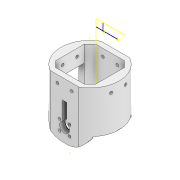
# Autodesk Inventor part: brazo_base_salvaculos.pt
Saved by Autodesk Inventor 2021 (Build 250183000, 183)
## iProperties
Created: 2021-03-15
Part Number: brazo_base_salvaculos.pt
Material: Plástico ABS
Document SubType Name: Modeling
Designer: Joaquín
Density: 1.06 g/cm^3
Appearance: Suave - Blanco
Author: Joaquín
Autodesk Inventor part; units mm, degrees
ref_plane "YZ Plane" through (0, 0, 0) normal (1, 0, 0) x (0, 1, 0)
ref_plane "XZ Plane" through (0, 0, 0) normal (0, 1, 0) x (-1, 0, 0)
ref_plane "XY Plane" through (0, 0, 0) normal (0, 0, 1) x (1, 0, 0)
sketch "Boceto4" plane through (0, 0, 0) normal (0, 1, 0) x (-1, 0, 0)
  line L0 (-22.5, 0) -> (-22.5, -16)
  line L1 (0, -22.5) -> (-16, -22.5)
  line L2 (-16, -22.5) -> (-22.5, -16)
  line L3 (0, -22.5) -> (16, -22.5)
  line L4 (22.5, 0) -> (22.5, -16)
  line L5 (22.5, -16) -> (16, -22.5)
  line L6 (22.5, 0) -> (22.5, 16)
  line L7 (0, 22.5) -> (16, 22.5)
  line L8 (16, 22.5) -> (22.5, 16)
  line L9 (0, 22.5) -> (-16, 22.5)
  line L10 (-22.5, 0) -> (-22.5, 16)
  line L11 (-22.5, 16) -> (-16, 22.5)
  line L12 (-16, 25) -> (16, 25)
  line L13 (25, 16) -> (25, -16)
  line L14 (16, -25) -> (-16, -25)
  line L15 (-25, -16) -> (-25, 16)
  line L16 (16, -25) -> (25, -16)
  line L17 (25, 16) -> (16, 25)
  line L18 (-25, 16) -> (-16, 25)
  line L19 (-25, -16) -> (-16, -25)
  point P0 (0, 0)
  dimension "d22" = 360
  constraints: 40 end point, 3 parallel, 1 horizontal, 1 perpendicular, 29 other
extrude "Extrusión2" add sketch "Boceto4" along normal blind 100
sketch "Boceto5" plane through (0, 0, 0) normal (0, -1, 0) x (1, 0, 0)
  circle A0 centre (0, 0) radius 32.5
  line L0 (-25, -16) -> (-25, 16) projected
  line L1 (-25, 16) -> (-16, 25) projected
  line L2 (-25, 16) -> (-16, 25)
  line L3 (-16, 25) -> (16, 25)
  line L4 (16, 25) -> (25, 16) projected
  line L5 (16, 25) -> (25, 16)
  line L6 (25, 16) -> (25, -16) projected
  line L7 (25, 16) -> (25, -16)
  line L8 (25, -16) -> (16, -25)
  line L9 (16, -25) -> (-16, -25) projected
  line L10 (16, -25) -> (-16, -25)
  line L11 (-16, -25) -> (-25, -16)
  line L12 (-25, -16) -> (-25, 16)
  constraints: 16 end point, 6 equal length, 1 centre point, 1 coincident, 1 horizontal, 1 perpendicular
sketch "Boceto7" plane through (-16, 0, 25) normal (0, 0, 1) x (1, 0, 0)
  line L0 (-9, 18) -> (-1.4121, 2.8243)
  line L1 (41, 0) -> (41, 100) projected
  line L2 (32, 0) -> (32, 100) projected
  line L3 (33.4121, 2.8243) -> (41, 18)
  line L4 (-9, 0) -> (-9, 100) projected
  line L5 (-19, 18) -> (-19, 0)
  line L6 (51, 18) -> (51, 0)
  line L7 (-9, 0) -> (-9, 10)
  line L8 (-9, 0) -> (-9, 100) projected
  line L9 (41, 0) -> (41, 10)
  line L10 (41, 10) -> (-9, 10)
  line L11 (-9, 10) -> (16, 10)
  ellipse E0 centre (16, 10) end of major axis (-9, 10) minor radius 10 (-1.4121, 2.8243) -> (33.4121, 2.8243) ccw
  line L12 (0, 0) -> (0, 100) projected
  line L13 (-19, 0) -> (16, 0)
  line L14 (16, 0) -> (51, 0)
  line L15 (32, 0) -> (0, 0) projected
  line L16 (-19, 18) -> (-19, 38)
  line L17 (51, 18) -> (51, 38)
  arc A0 (-19, 38) -> (-9, 18) centre (10.8998, 40.4499) ccw
  arc A1 (41, 18) -> (51, 38) centre (21.1002, 40.4499) ccw
  point P0 (32, 2.3163)
  dimension "d53" = 10
  dimension "d54" = 10
  dimension "d55" = 25
  dimension "d58" = 20
  dimension "d59" = 20
  dimension "d60" = 30
  dimension "d61" = 30
  constraints: 24 end point, 4 point on circle, 4 point on line, 2 centre point, 2 horizontal, 2 vertical, 1 coincident, 1 collinear, 1 midpoint, 5 other
  measures "d53" distance of L7.end L4.start
  measures "d54" distance of L1.start L9.end
  measures "d55" distance of L7.end L11.end
  measures "d58" distance of L5.start L16.end
  measures "d59" distance of L6.start L17.end
  measures "d60" radius of A0
  measures "d61" radius of A1
extrude "Extrusión4" add sketch "Boceto5" against normal blind 100
extrude "Extrusión8" cut sketch "Boceto7" against normal mid plane 200 contours L0 L10 L4 | L4 L13 L5 L16 A0 | L0 E0 L12 L13 L4 L10 | E0 L13 L12 | E0 L2 L14 | E0 L3 L10 L1 L14 L2 | L3 L1 L10 | L1 A1 L17 L6 L14
sketch "Boceto10" plane through (-16, 100, -22.5) normal (0, 0, 1) x (1, 0, 0)
  line L0 (0, 0) -> (8, 0)
  line L1 (0, 0) -> (32, 0) projected
  line L2 (8, 0) -> (8, -8)
  circle A0 centre (8, -8) radius 1.5
  line L3 (32, -97.6837) -> (32, 0) projected
  line L4 (32, 0) -> (24, 0)
  line L5 (24, 0) -> (24, -8)
  circle A1 centre (24, -8) radius 1.5
  point P0 (16, -100)
  dimension "d95" = 8
  dimension "d96" = 8
  dimension "d97" = 3
  dimension "d98" = 8
  dimension "d99" = 8
  dimension "d100" = 3
  constraints: 8 end point, 2 centre point, 2 coincident, 2 perpendicular, 2 point on line
  measures "d95" distance of L0.start L0.end
  measures "d96" distance of L0.end L2.end
  measures "d97" diameter of A0
  measures "d98" distance of L1.end L4.end
  measures "d99" distance of L4.end L5.end
  measures "d100" diameter of A1
extrude "Extrusión12" cut sketch "Boceto10" along normal mid plane 200
sketch "Boceto11" plane through (22.5, 100, -16) normal (-1, 0, 0) x (0, 0, 1)
  circle A0 centre (8, -8) radius 1.5
  circle A1 centre (24, -8) radius 1.5
  point P0 (16, -100)
  point P1 (0, 0)
  point P2 (32, 0)
  constraints: 2 centre point
extrude "Extrusión13" cut sketch "Boceto11" against normal mid plane 200
sketch "Boceto14" plane through (0, 100, 0) normal (0, 1, 0) x (1, 0, 0)
  point P0 (0, 0)
sketch "Boceto15" plane through (-16, 100, -22.5) normal (0, 0, 1) x (1, 0, 0)
  line L0 (13, -81) -> (10, -81) projected
  line L1 (22, -69) -> (19, -69) projected
  arc A0 (32, -94.1587) -> (0, -94.1587) centre (16, -75.1663) ccw
  circle A1 centre (16, -75.1663) radius 20
  line L2 (0, -97.6837) -> (0, 0) projected
  line L3 (0, -87.1663) -> (0, -97.6837)
  line L4 (32, -97.6837) -> (32, 0) projected
  line L5 (32, -87.1663) -> (32, -97.6837)
  ellipse E0 centre (16, -90) end of major axis (41, -90) minor radius 10 (-1.4121, -97.1757) -> (0, -97.6837) ccw projected
  line L6 (0, -110.3048) -> (31.8425, -110.6904)
  line L7 (0, -87.1663) -> (-17.9607, -87.1663)
  line L8 (32, -87.1663) -> (50.1944, -87.1663)
  line L9 (50.1944, -87.1663) -> (31.8425, -110.6904)
  line L10 (-17.9607, -87.1663) -> (0, -110.3048)
  point P0 (10, -69)
  point P1 (0, -94.1587)
  point P2 (-5.742, -87.1663)
  point P3 (37.742, -87.1663)
  constraints: 14 end point, 4 point on circle, 3 point on line, 2 centre point, 2 collinear, 2 horizontal, 1 coincident, 1 other
extrude "Extrusión16" cut sketch "Boceto15" along normal mid plane 1000 contours A0 L8 L9 L6 L10 L7 L2 A1 L4
sketch "Boceto16" plane through (16, 5.8413, -22.5) normal (-1, 0, 0) x (0, 0, 1)
  line L0 (0, 6.9924) -> (0, 94.1587) projected
  line L1 (-5.7887, 0) -> (-5.7887, 6.9924) projected
  line L2 (0, 6.9924) -> (-5.7887, 6.9924)
  line L3 (-5.7887, 6.9924) -> (-5.7887, -0.349)
  line L4 (-5.7887, -0.349) -> (0, 0)
  line L5 (0, 0) -> (0, 6.9924) projected
  line L6 (0, 0) -> (0, 6.9924)
  line L7 (50.7887, 6.9924) -> (50.7887, 0) projected
  line L8 (50.7887, 6.9924) -> (50.7887, 0)
  line L9 (45, 0) -> (45, 6.9924) projected
  line L10 (50.7887, 0) -> (45, 0)
  line L11 (45, 0) -> (45, 6.9924)
  line L12 (45, 6.9924) -> (50.7887, 6.9924)
  point P0 (22.5, -5.8413)
  constraints: 16 end point, 3 collinear, 3 perpendicular, 1 vertical
extrude "Extrusión17" cut sketch "Boceto16" along normal mid plane 1000
sketch "Boceto17" plane through (16, 12.8337, 22.5) normal (0, 0, 1) x (1, 0, 0)
  line L0 (-32, 0) -> (-37.742, 0) projected
  line L1 (-32, 0) -> (-43.1416, 0)
  line L2 (-43.1416, 0) -> (-43.4949, -15.0016)
  line L3 (-43.4949, -15.0016) -> (-30.7161, -15.0016)
  line L4 (0, 0) -> (-32, 0) projected
  line L5 (-30.7161, -15.0016) -> (-32, 0)
  line L6 (5.742, 0) -> (0, 0) projected
  arc A0 (0, -6.9924) -> (5.742, 0) centre (-16, 12) ccw projected
  line L7 (0, 0) -> (0, -6.9924)
  line L8 (0, -6.9924) -> (6.855, -6.9924)
  line L9 (6.855, -6.9924) -> (5.742, 0)
  line L10 (5.742, 0) -> (0, 0)
  point P0 (-16, -12.8337)
  constraints: 16 end point, 2 parallel, 1 horizontal, 1 perpendicular, 1 vertical
extrude "Extrusión18" cut sketch "Boceto17" along normal mid plane 1000
sketch "Boceto18" plane through (-6.268, 5.8413, 28.2887) normal (0, 1, 0) x (1, 0, 0)
  circle A0 centre (82.4953, 58.0678) radius 132.1939
  point P0 (6.268, 28.2887)
  constraints: 1 centre point
extrude "Extrusión19" cut sketch "Boceto18" against normal blind 1000
sketch "Boceto19" plane through (-16, 12.8337, -28.2887) normal (0, 0, 1) x (1, 0, 0)
  line L0 (0, 0) -> (32, 0) projected
  line L1 (0, 0) -> (32.4296, 0)
  line L2 (32.4296, 0) -> (32.4296, -12.309)
  line L3 (32.4296, -12.309) -> (0, -12.309)
  line L4 (0, -12.309) -> (0, 0)
  point P0 (16, -12.8337)
  constraints: 8 end point, 2 parallel, 1 horizontal, 1 perpendicular
extrude "Extrusión20" cut sketch "Boceto19" against normal mid plane 1000
sketch "Boceto21" plane through (16, 100, 22.5) normal (0, 0, -1) x (-1, 0, 0)
  line L0 (32, -87.1663) -> (32, 0) projected
  circle A0 centre (16, -72.1663) radius 5.5
  circle A1 centre (21.5984, -66.4516) radius 1.5
  circle A2 centre (10.4016, -66.4516) radius 1.5
  circle A3 centre (10.4016, -77.881) radius 1.5
  circle A4 centre (21.5984, -77.881) radius 1.5
  line L1 (16, -72.1663) -> (16, -66.6663)
  line L2 (18.5, -66.6663) -> (18.5, -67.2673)
  line L3 (13.5, -66.6663) -> (13.5, -67.2673)
  line L4 (13.5, -66.6663) -> (13.5, -46.6663)
  line L5 (13.5, -46.6663) -> (18.5, -46.6663)
  line L6 (18.5, -46.6663) -> (18.5, -66.6663)
  line L7 (13.5, -66.6663) -> (18.5, -66.6663)
  point P0 (16, -100)
  point P1 (0, -87.1663)
  dimension "d151" = 20
  dimension "d152" = 5
  constraints: 14 end point, 5 centre point, 3 point on circle, 2 perpendicular, 2 vertical, 1 collinear
  measures "d151" distance of L3.start L4.end
  measures "d152" distance of L4.end L5.end
extrude "Extrusión21" cut sketch "Boceto21" along normal mid plane 1000 contours A0 | A0 L7 L2 | L3 L7 A0 | A1 | A2 | A3 | A4
sketch "Boceto22" plane through (-2.5, 33.3337, 22.5) normal (0, -1, 0) x (1, 0, 0)
  point P0 (2.5, -22.5)
sketch "Boceto23" plane through (-2.5, 33.3337, 22.5) normal (0, -1, 0) x (1, 0, 0)
  arc A0 (0, -54.9037) -> (5, -54.9037) centre (2.5, -22.5) ccw projected
  line L0 (5, -54.9037) -> (5, -46.9037)
  line L1 (5, -46.9037) -> (0, -46.9037)
  line L2 (0, -45) -> (0, -54.9037) projected
  line L3 (0, -54.9037) -> (0, -46.9037)
  line L4 (5, -54.9037) -> (5.1163, -56.9374)
  line L5 (5.1163, -56.9374) -> (0, -61.3035)
  line L6 (0, -61.3035) -> (0, -54.9037)
  dimension "d155" = 8
  constraints: 12 end point, 2 perpendicular, 1 collinear, 1 point on line, 1 vertical
  measures "d155" distance of L0.start L0.end
extrude "Extrusión22" cut sketch "Boceto23" against normal blind 20
sketch "Boceto24" plane through (-2.5, 33.3337, 22.5) normal (0, -1, 0) x (1, 0, 0)
  line L0 (0, 9.9037) -> (0, 0) projected
  line L1 (0, 9.9037) -> (0, 1.9037)
  line L2 (0, 1.9037) -> (5, 1.9037)
  line L3 (5, 0) -> (5, 9.9037) projected
  line L4 (5, 9.9037) -> (5, 1.9037)
  arc A0 (5, 9.9037) -> (0, 9.9037) centre (2.5, -22.5) ccw
  dimension "d164" = 8
  constraints: 6 end point, 2 point on circle, 2 point on line, 1 centre point, 1 coincident, 1 collinear, 1 perpendicular
  measures "d164" distance of L0.start L1.end
extrude "Extrusión23" cut sketch "Boceto24" against normal blind 20
chamfer "Chaflán3" distance 2 angle 45 6 edges at (2.5, 43.0332, -32.4037) (0, 53.3337, -32.5) (-2.5, 43.0332, -32.4037) (0, 53.3337, 32.5) (-2.5, 43.0332, 32.4037) (2.5, 43.0332, 32.4037)
sketch "Boceto25" plane through (-16, 100, -22.5) normal (0, 0, 1) x (1, 0, 0)
  circle A0 centre (24, -8) radius 1.5 projected
  circle A1 centre (8, -8) radius 1.5 projected
  line L0 (24, -8) -> (8, -8)
  line L1 (8, -8) -> (0, -8)
  line L2 (0, -87.1663) -> (0, 0) projected
  line L3 (8, -8) -> (8, 0)
  line L4 (0, 0) -> (32, 0) projected
  point P0 (16, -100)
  constraints: 6 end point, 3 point on line, 1 horizontal, 1 perpendicular
sketch "Boceto26" plane through (0, 100, 0) normal (0, 1, 0) x (1, 0, 0)
  circle A0 centre (0, 0) radius 51.8697
  constraints: 1 centre point, 1 coincident
extrude "Extrusión24" cut sketch "Boceto26" against normal blind 25
sketch "Boceto27" plane through (-16, 12.8337, -22.5) normal (0, 0, 1) x (1, 0, 0)
  point P0 (16, -12.8337)
sketch "Boceto28" plane through (-16, 12.8337, -22.5) normal (0, 0, 1) x (1, 0, 0)
  circle A0 centre (24, 54.1663) radius 1.5
  circle A1 centre (8, 54.1663) radius 1.5
  point P0 (16, -12.8337)
  point P1 (0, 62.1663)
  constraints: 2 centre point
extrude "Extrusión25" cut sketch "Boceto28" against normal mid plane 250
sketch "Boceto29" plane through (-22.5, 13, 16) normal (1, 0, 0) x (0, 0, -1)
  line L0 (0, 62) -> (-1.3246, 65.4001)
  circle A0 centre (8, 54) radius 1.5
  circle A1 centre (24, 54) radius 1.5
  point P0 (16, -13)
  dimension "d178" = 3
  constraints: 2 centre point, 2 end point
  measures "d178" diameter of A1
extrude "Extrusión26" cut sketch "Boceto29" against normal mid plane 250
sketch "Boceto30" plane through (16, 12.8337, 22.5) normal (0, 0, -1) x (-1, 0, 0)
  arc A0 (13.5, 19.899) -> (18.5, 19.899) centre (16, 15) ccw projected
  circle A1 centre (16, 15) radius 5.5
  circle A2 centre (21.5984, 20.7147) radius 1.5 projected
  circle A3 centre (21.5984, 20.7147) radius 1.5
  circle A4 centre (10.4016, 20.7147) radius 1.5 projected
  circle A5 centre (10.4016, 20.7147) radius 1.5
  circle A6 centre (10.4016, 9.2853) radius 1.5 projected
  circle A7 centre (10.4016, 9.2853) radius 1.5
  circle A8 centre (21.5984, 9.2853) radius 1.5 projected
  circle A9 centre (21.5984, 9.2853) radius 1.5
  point P0 (16, -12.8337)
  constraints: 5 centre point, 5 coincident
sketch "Boceto31" plane through (-22.5, 13, 16) normal (1, 0, 0) x (0, 0, -1)
  line L0 (0, 0) -> (-15, 0)
  line L1 (-6.5, -0.1663) -> (-0.0832, -0.1663) projected
  line L2 (-0.0832, -0.1663) -> (0, 14.8335)
  line L3 (0, 0) -> (0, 62) projected
  line L4 (0, 14.8335) -> (32.0005, 14.8335)
  line L5 (32.0005, 14.8335) -> (32.0005, -2.3948)
  line L6 (32, 0) -> (32, 62) projected
  line L7 (32.0005, -2.3948) -> (0, -2.3948)
  line L8 (0, -2.3948) -> (0, 0)
  point P0 (16, -13)
  dimension "d181" = 15
  dimension "d182" = 15
  constraints: 12 end point, 3 perpendicular, 1 parallel, 1 point on line
  measures "d181" distance of L0.start L0.end
  measures "d182" distance of L1.end L2.end
extrude "Extrusión27" cut sketch "Boceto31" against normal mid plane 1010 contours L3 L4 L5 L7 L8
sketch "Boceto32" plane through (-28.2884, 27.8335, -16.0005) normal (0, 0, 1) x (1, 0, 0)
  line L0 (0, 0) -> (5.7889, 0) projected
  line L1 (5.7889, 0) -> (-1.1993, 0)
  line L2 (-1.1993, 0) -> (-1.1993, -18.8213)
  line L3 (-1.1993, -18.8213) -> (63.7821, -18.8213)
  line L4 (-1.1993, 0) -> (77.5242, 0)
  line L5 (77.5242, 0) -> (63.7821, -18.8213)
  point P0 (28.2884, -27.8335)
  constraints: 10 end point, 2 perpendicular, 1 collinear, 1 point on line
extrude "Extrusión28" cut sketch "Boceto32" against normal blind 5
sketch "Boceto33" plane through (28.2887, 27.8335, 16) normal (0, 0, -1) x (-1, 0, 0)
  line L0 (0, 0) -> (-4.0296, 0) projected
  line L1 (-4.0296, 0) -> (64.5612, 0)
  line L2 (64.5612, 0) -> (65.7148, -27.0644)
  line L3 (65.7148, -27.0644) -> (-2.0148, -25.6546)
  line L4 (-2.0148, -25.6546) -> (-4.0296, 0)
  point P0 (28.2887, -27.8335)
  constraints: 8 end point, 1 horizontal
extrude "Extrusión29" cut sketch "Boceto33" against normal blind 5
sketch "Boceto34" plane through (-16, 12.8337, -22.5) normal (0, -1, 0) x (1, 0, 0)
  line L0 (0, 0) -> (0, -5.7887)
  line L1 (0, -5.7887) -> (-5, -5.7887)
  line L2 (32, 50.7887) -> (37, 50.7887)
  line L3 (0, -5.7887) -> (37, -5.7887)
  line L4 (32, 50.7887) -> (-5, 50.7887)
  arc A0 (37, 50.7887) -> (-5, 50.7887) centre (16, 22.5) ccw
  arc A1 (-5, -5.7887) -> (37, -5.7887) centre (16, 22.5) ccw
  point P0 (32, 45)
  dimension "d189" = 5
  dimension "d190" = 5
  constraints: 10 end point, 4 point on circle, 2 centre point, 2 horizontal, 1 coincident, 1 perpendicular, 1 vertical
  measures "d189" distance of L0.end L1.end
  measures "d190" distance of L2.start L2.end
sketch "Boceto35" plane through (16, 12.8337, 22.5) normal (0, 0, -1) x (-1, 0, 0)
  line L0 (0, 0) -> (32, 0) projected
  line L1 (-8.8042, 14.9998) -> (-1.5, 14.9998) projected
  line L2 (40.8042, 14.9998) -> (40.8042, 4.7748) projected
  line L3 (-8.8042, 4.7748) -> (-8.8042, 14.9998) projected
  arc A0 (-8.8042, 14.9998) -> (16, 0) centre (14.1387, 24.9306) ccw
  arc A1 (16, 0) -> (40.8042, 14.9998) centre (17.8613, 24.9306) ccw
  line L4 (-8.8042, 14.9998) -> (-15.703, 14.2215)
  line L5 (-15.703, 14.2215) -> (-20.1615, -19.8181)
  line L6 (-20.1615, -19.8181) -> (61.4705, -19.1747)
  line L7 (61.4705, -19.1747) -> (55.8092, 13.853)
  line L8 (55.8092, 13.853) -> (40.8042, 14.9998)
  point P0 (16, -12.8337)
  constraints: 10 end point, 4 point on circle, 2 centre point, 1 midpoint
extrude "Extrusión30" cut sketch "Boceto35" against normal mid plane 200 contours A0 A1 L8 L7 L6 L5 L4
extrude "Extrusión31" cut sketch "Boceto34" against normal blind 200
sketch "Boceto36" plane through (-22.5, 75, 16) normal (1, 0, 0) x (0, 0, -1)
  line L0 (0, -47.1665) -> (0, 0) projected
  line L1 (0, -47.1665) -> (0, -18.2089)
  line L2 (0, -18.2089) -> (32, -18.2089)
  line L3 (32, -47.1665) -> (32, 0) projected
  line L4 (32, -47.1665) -> (37.0005, -47.1665) projected
  line L5 (32, -47.1665) -> (32, -18.2089)
  line L6 (0, -47.1665) -> (32, -47.1665) projected
  line L7 (32, -47.1665) -> (0, -47.1665)
  point P0 (16, -75)
  constraints: 8 end point, 2 perpendicular, 2 point on line, 1 horizontal
extrude "Extrusión32" cut sketch "Boceto36" against normal blind 20
